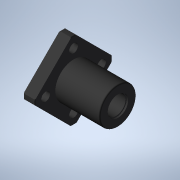
# Autodesk Inventor part: C-LHFS10
Saved by Autodesk Inventor 2021 (Build 250183000, 183)
## iProperties
Created: 2025-02-22
Part Number: C-LHFS10
Material: Generic
Catalog Web Link: www.cadenas.de
Description: C-LHFR, C-LHFS, C-LHFC, C-LHFRM, C-LHFSM, C-LHFCM,C-LHFCF-N,C-LHFCMF-N-Flanged Linear Bushings - Standard - C-VALUE Single Type
Vendor: MISUMI
Document SubType Name: Modeling
Designer: psAdmin
Manufacturer: MISUMI
Mass: 8.72893 g
Surface Area: 50.0314 cm^2
Volume: 8.72893 cm^3
Density: 1 g/cm^3
Appearance: PSOLRGB-175-175-175
Category: PARTsolutions
Company: MISUMI
Title: C-LHFS10
Author: Cadenas PARTsolutions
Comments: Flanged Linear Bushings - Standard - C-VALUE Single Type
PSOL_IDENT_0: {$CADENAS_DATA/23d-libs/misumi/metric/04_linear_bushings/c_lhfr.prj},228 {VTYP=3D},{NB=C-LHFS10},{LI
PSOL_IDENT_1: NA=C-LHFS10},{NN=C-LHFR, C-LHFS, C-LHFC, C-LHFRM, C-LHFSM, C-LHFCM,C-LHFCF-N,C-LHFCMF-N},{DATE=16.08
PSOL_IDENT_2: .2023 02:43:51},{GEOMDATE=03.08.2023 03:48:35},{VERSION=},{LINEID=60},{WBVAR=SS,TS,ST},{WBNUMERIC=}
PSOL_IDENT_3: {NB=C-LHFS10},{LINA=C-LHFS10},{KT=DUMMY},{PN=C-LHFS10},{TYPE=C-LHFS},{SS=S},{SSALG='S','Standard Sp
PSOL_IDENT_4: ecifications','HT','High Temperature Specification'},{TS=S},{TSALG='R', 'Round Flange', 'S', 'Square
PSOL_IDENT_5: Flange', 'C', '2 - Flats Flange'},{ST=},{STALG='', '-', 'ENP', 'Electroless Nickel Plating'},{DDRR=
PSOL_IDENT_6: 10},{D=19},{L=29},{H=40},{T=6},{DD=4.5},{DD1=7.5},{TT=4.1},{PCD=29},{PCDFX=29},{W=30},{WFX=30},{F=0}
PSOL_IDENT_7: ,{FFX=0},{A=0},{AFX=29},{K=0},{KFX=25},{BR=4},{TIFF=2},{R=0.6},{C=0.30},{DD2=10.6},{DD3=11.2},{Y=0.7
PSOL_IDENT_8: },{Z=0.35}
NB: C-LHFS10
NN: C-LHFR, C-LHFS, C-LHFC, C-LHFRM, C-LHFSM, C-LHFCM,C-LHFCF-N,C-LHFCMF-N
NT: Flanged Linear Bushings - Standard - C-VALUE Single Type
NBSYN: $PN.
LINA: C-LHFS10
CATALOG: Misumi
PN: C-LHFS10
TYPE: C-LHFS
SS: Standard Specifications
TS: Square Flange
ST: -
DDRR: 10
D: 19
L: 29
H: 40
T: 6
DD: 4.5
DD1: 7.5
TT: 4.1
PCD: 29
W: 30
F: 0
A: 0
K: 0
SUPPLIER: MISUMI
ARTICLENO: C-LHFS10
BOMINFO: C-LHFS10
CREATOR: CADENAS GmbH
Autodesk Inventor part; units mm, degrees
sketch "Sketch_1" plane through (0, 0, 0) normal (0, 0, 1) x (1, 0, 0)
  line L0 (29, 0) -> (0, 0)
  line L1 (0, 5.3) -> (0.7, 5.3)
  line L2 (0.7, 5.3) -> (0.7, 5.6)
  line L3 (0.7, 5.6) -> (1.05, 5.6)
  line L4 (1.05, 5.6) -> (1.05, 5)
  line L5 (1.05, 5) -> (27.95, 5)
  line L6 (27.95, 5) -> (27.95, 5.6)
  line L7 (27.95, 5.6) -> (28.3, 5.6)
  line L8 (28.3, 5.6) -> (28.3, 5.3)
  line L9 (28.3, 5.3) -> (29, 5.3)
  line L10 (29, 5.3) -> (29, 8.9)
  arc A0 (29, 8.9) -> (28.4, 9.5) centre (28.4, 8.9) ccw
  line L11 (28.4, 9.5) -> (6, 9.5)
  line L12 (6, 9.5) -> (6, 19.7)
  line L13 (6, 19.7) -> (5.7, 20)
  line L14 (5.7, 20) -> (0.3, 20)
  line L15 (0.3, 20) -> (0, 19.7)
  line L16 (0, 19.7) -> (0, 5.3)
  constraints: 34 end point, 2 point on circle, 1 centre point
revolve "Revolution1" add sketch "Sketch_1" angle 360 about axis through (29, 0, 0) along (1, 0, 0)
sketch "Sketch_2" plane through (0, 0, 0) normal (1, 0, 0) x (0, 1, 0)
  line L0 (-30, 30) -> (-30, -30)
  line L1 (-30, -30) -> (30, -30)
  line L2 (30, -30) -> (30, 30)
  line L3 (30, 30) -> (-30, 30)
  line L4 (-1.2132, 20) -> (-20, 1.2132)
  line L5 (-20, 1.2132) -> (-20, -1.2132)
  line L6 (-20, -1.2132) -> (-1.2132, -20)
  line L7 (-1.2132, -20) -> (1.2132, -20)
  line L8 (1.2132, -20) -> (20, -1.2132)
  line L9 (20, -1.2132) -> (20, 1.2132)
  line L10 (20, 1.2132) -> (1.2132, 20)
  line L11 (1.2132, 20) -> (-1.2132, 20)
  constraints: 24 end point
extrude "Extrusion1" cut sketch "Sketch_2" along normal blind 6
sketch "Sketch3" plane through (0, 0, 0) normal (-1, 0, 0) x (0, 0, 1)
  point P0 (0, 14.5)
hole "Hole1" at (0, 14.5, 0) direction (1, 0, 0) diameter 4.5 depth 6 counterbore diameter 7.5 counterbore depth 4.1
sketch "Sketch4" plane through (0, 0, 0) normal (-1, 0, 0) x (0, 0, 1)
  point P0 (0, -14.5)
hole "Hole2" at (0, -14.5, 0) direction (1, 0, 0) diameter 4.5 depth 6 counterbore diameter 7.5 counterbore depth 4.1
sketch "Sketch5" plane through (0, 0, 0) normal (-1, 0, 0) x (0, 0, 1)
  point P0 (-14.5, 0)
hole "Hole3" at (0, 0, -14.5) direction (1, 0, 0) diameter 4.5 depth 6 counterbore diameter 7.5 counterbore depth 4.1
sketch "Sketch6" plane through (0, 0, 0) normal (-1, 0, 0) x (0, 0, 1)
  point P0 (14.5, 0)
hole "Hole4" at (0, 0, 14.5) direction (1, 0, 0) diameter 4.5 depth 6 counterbore diameter 7.5 counterbore depth 4.1
ref_plane "Combination_Module_XY" through (0, 0, 0) normal (1, 0, 0) x (0, 0, -1)
ref_plane "Combination_Module_YZ" through (0, 0, 0) normal (0, 0, -1) x (0, 1, 0)
ref_plane "Combination_Module_ZX" through (0, 0, 0) normal (0, 1, 0) x (1, 0, 0)
body "Solid1"
